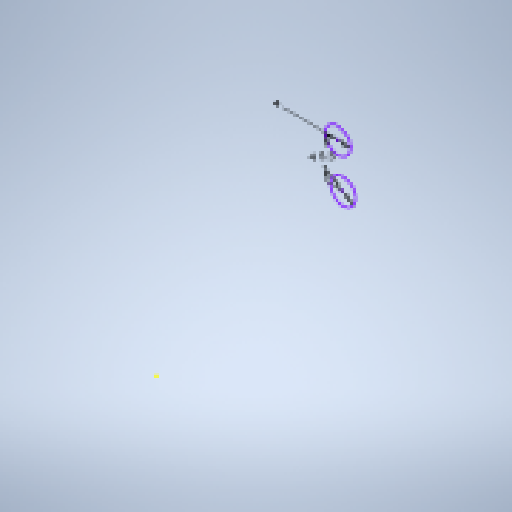
# Autodesk Inventor part: SlideStopBearingHolder
Saved by Autodesk Inventor 2023 (Build 270158000, 158)
## iProperties
Created: 2022-10-07
Part Number: SlideStopBearingHolder
Material: Generic
Document SubType Name: Modeling
Designer: deli
Density: 1 g/cm^3
Appearance: Default
Author: deli
Autodesk Inventor part; units mm, degrees
ref_plane "YZ Plane" through (0, 0, 0) normal (1, 0, 0) x (0, 1, 0)
ref_plane "XZ Plane" through (0, 0, 0) normal (0, 1, 0) x (-1, 0, 0)
ref_plane "XY Plane" through (0, 0, 0) normal (0, 0, 1) x (1, 0, 0)
sketch "Sketch1" plane through (0, 0, 0) normal (0, 0, 1) x (1, 0, 0)
  circle A0 centre (26.4431, 48.9117) radius 2
  circle A1 centre (26.4431, 42.4117) radius 2
  line L0 (16.4431, 54.1617) -> (32.9431, 54.1617)
  line L1 (32.9431, 54.1617) -> (32.9431, 37.1617)
  line L2 (32.9431, 37.1617) -> (16.4431, 37.1617)
  line L3 (16.4431, 37.1617) -> (16.4431, 54.1617)
  point P0 (0, 0)
  dimension "d0" = 4
  dimension "d1" = 4
  dimension "d2" = 6.5
  dimension "d4" = 17
  dimension "d5" = 5.25
  dimension "d6" = 6.5
  dimension "d7" = 6.5
  dimension "d8" = 10
  constraints: 8 end point, 2 centre point, 2 parallel, 1 horizontal, 1 perpendicular
  measures "d0" diameter of A0
  measures "d1" diameter of A1
  measures "d2" distance of A0.centre A1.centre
  measures "d4" distance of L0.end L1.end
  measures "d5" distance from line of L0 A0.centre
  measures "d6" distance from line of L1 A0.centre
  measures "d7" distance from line of L1 A1.centre
  measures "d8" distance from line of A0.centre L3
extrude "Extrusion1" add sketch "Sketch1" along normal blind 6.35
sketch "Sketch2" plane through (16.4431, 37.1617, 0) normal (-1, 0, 0) x (0, 0, 1)
  circle A0 centre (3.175, 8.5) radius 1.25
  line L0 (0, 17) -> (6.35, 0) construction
  line L1 (0, 0) -> (6.35, 0) construction
  line L2 (0, 0) -> (6.35, 17) construction
  point P0 (0, -37.1617)
  dimension "d11" = 2.5
  constraints: 4 end point, 2 coincident, 2 midpoint, 1 centre point
  measures "d11" diameter of A0
extrude "Extrusion2" cut sketch "Sketch2" against normal blind 8
thread "Thread1" size "M3x0.5" class "6H" standard "ANSI Metric M Profile" full length
fillet "Fillet1" radius 4 4 edges at (16.4431, 54.1617, 3.175) (32.9431, 54.1617, 3.175) (16.4431, 37.1617, 3.175) (32.9431, 37.1617, 3.175)
equation "\"d5\" = -0.5 * d2 + 0.5 * d4"
equation "\"d7\" = d6"
body "Solid1"
